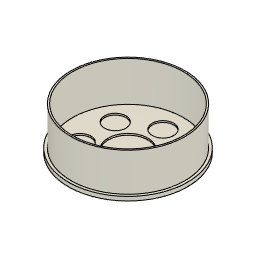
Basis_Vitrine (Autodesk Fusion 360 design; units mm, degrees)
Autodesk Fusion 360 part; units mm, degrees
sketch "Skizze1" plane through (0, 0, 0) normal (0, 1, 0) x (1, 0, 0)
  circle A0 centre (0, 0) radius 71.7
  circle A1 centre (0, 0) radius 68.7
  circle A2 centre (0, 0) radius 25
  circle A3 centre (0, 44) radius 13.5
  circle A4 centre (-38.1051, 22) radius 13.5
  circle A5 centre (-38.1051, -22) radius 13.5
  circle A6 centre (0, -44) radius 13.5
  circle A7 centre (38.1051, -22) radius 13.5
  circle A8 centre (38.1051, 22) radius 13.5
  dimension "d2" = 143.4
  dimension "d3" = 3
  dimension "d4" = 50
  dimension "d11" = 27
  dimension "d13" = 360
  dimension "d17" = 44
  dimension "d25" = 44
  constraint coincident A0.centre A1.centre
  constraint concentric A0 A1
  measures "d2" diameter of A0
  measures "d3" distance of A0 A1
  measures "d4" diameter of A2
  measures "d11" diameter of A3
  measures "d17" distance of A0.centre A3.centre
  measures "d25" distance of A3.centre A8.centre
extrude "Extrusion1" add sketch "Skizze1" along normal blind 2 contours A1 | A3 | A4 | A5 | A6 | A7 | A8 makes body 1
extrude "Extrusion2" add sketch "Skizze1" against normal blind 1 contours A0 | A1 | A2 | A3 | A4 | A5 | A6 | A7 | A8 bodies 1
extrude "Extrusion3" add sketch "Skizze1" along normal blind 60 contours A0 bodies 1
extrude "Extrusion4" cut sketch "Skizze1" against normal blind 2 from surface at 2 contours A3 | A4 | A5 | A6 | A7 | A8 bodies 1
sketch "Skizze2" plane through (0, 60, 0) normal (0, 1, 0) x (-1, 0, 0)
  circle A0 centre (0, 0) radius 68.7
  circle A1 centre (0, 0) radius 71.7
  circle A2 centre (0, 0) radius 68.3
  circle A3 centre (0, 0) radius 63.7
  dimension "d19" = -0.4
  dimension "d22" = -5
extrude "Extrusion5" add sketch "Skizze2" along normal blind 4 separate body contours A0 | A1 | A2 | A3 makes body 2
extrude "Extrusion6" add sketch "Skizze2" against normal blind 5 contours A2 bodies 2
sketch "Skizze3" plane through (0, -1, 0) normal (0, -1, 0) x (1, 0, 0)
  circle A0 centre (0, 0) radius 71.7
  circle A1 centre (0, 0) radius 75
  dimension "d26" = 150
  constraint coincident A0.centre A1.centre
  measures "d26" diameter of A1
extrude "Extrusion7" add sketch "Skizze3" along normal blind 5 contours A0 | A1 bodies 1
extrude "Extrusion8" cut 7 faces at (36.4978, 0, -25.6989) (3.6941, 0, -49.6839) (-6.7759, 0, 1.242) (-46.8549, 0, -23.9971) (-34.6344, 0, 25.418) (-1.9803, 0, 52.6763) (42.9135, 0, 25.5182) along direction (0, -1, 0) blind 5 on bodies 1 bodies 1
extrude "Extrusion9" cut 1 faces at (26.9574, 2, -46.6916) along direction (0, -1, 0) blind 5 on bodies 1 bodies 1
move_face "Flächen versetzen1" offset -1 1 faces at (68.6146, 39, 3.4244) on bodies 1
extrude "Extrusion10" cut 1 faces at (-22.538, 60, -67.176) along direction (0, -1, 0) blind 13 on bodies 1 bodies 1
hidden bodies 2
equation "Durchmesser = Plexidurchmesser - 3 mm - 3 mm - 0.6 mm"
equation "d2 = Durchmesser"
equation "Plexidurchmesser = 150 mm"
named bodies: "Base", "Deckel"
